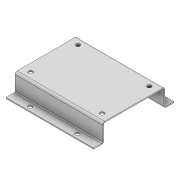
# Autodesk Inventor part: BaseMotor
Saved by Autodesk Inventor 2021 (Build 250183000, 183)
## iProperties
Created: 2021-08-18
Part Number: BaseMotor
Material: Generic
Document SubType Name: Sheet Metal
Designer: Santiago Suárez
Density: 1 g/cm^3
Sheet Metal Rule: Default_mm
Appearance: Default
Author: Santiago Suárez
Autodesk Inventor part; units mm, degrees
ref_plane "YZ Plane" through (0, 0, 0) normal (1, 0, 0) x (0, 1, 0)
ref_plane "XZ Plane" through (0, 0, 0) normal (0, 1, 0) x (-1, 0, 0)
ref_plane "XY Plane" through (0, 0, 0) normal (0, 0, 1) x (1, 0, 0)
sketch "Sketch1" plane through (0, 0, 0) normal (0, 1, 0) x (-1, 0, 0)
  line L0 (130, 92.5) -> (-130, 92.5)
  line L1 (-130, 92.5) -> (-130, -92.5)
  line L2 (-130, -92.5) -> (130, -92.5)
  line L3 (130, -92.5) -> (130, 92.5)
  point P0 (0, 0)
  dimension "d0" = 260
  dimension "d1" = 185
  dimension "d2" = 92.5
  dimension "d29" = 130
  measures "d0" distance of L0.start L0.end
  measures "d1" distance of L2.end L0.start
  measures "d2" distance from line of L0 point (0, 0)
  measures "d29" distance from line of L3 point (0, 0)
extrude "Plate1" add sketch "Sketch1" along normal blind 3.175
sketch "Sketch2" plane through (130, 3.175, 89.325) normal (0, 0, 1) x (1, 0, 0)
  line L0 (-260, 0) -> (0, 0)
  line L1 (0, 0) -> (0, 55)
  line L2 (0, 55) -> (-260, 55)
  line L3 (-260, 55) -> (-260, 0)
  constraints: 6 end point, 1 horizontal, 1 perpendicular, 1 vertical
edge flange "Flange1" height 55 angle 90 thickness 3.175 bend radius 3.175 thickness toward (0, 0, 1) relief straight relief width 3.175 relief depth 1.5875 edges at (0, 3.175, 92.5) wall of the first edge with corners at (-130, 3.175, 89.325) (130, 3.175, 89.325) (130, -51.825, 89.325) (-130, -51.825, 89.325)
bend "Bend1"
corner "Corner1"
sketch "Sketch3" plane through (-130, 3.175, -89.325) normal (0, 0, -1) x (-1, 0, 0)
  line L0 (-260, 0) -> (0, 0)
  line L1 (0, 0) -> (0, 55)
  line L2 (0, 55) -> (-260, 55)
  line L3 (-260, 55) -> (-260, 0)
  constraints: 6 end point, 1 horizontal, 1 perpendicular, 1 vertical
edge flange "Flange2" height 55 angle 90 thickness 3.175 bend radius 3.175 thickness toward (0, 0, -1) relief straight relief width 3.175 relief depth 1.5875 edges at (0, 3.175, -92.5) wall of the first edge with corners at (130, 3.175, -89.325) (-130, 3.175, -89.325) (-130, -51.825, -89.325) (130, -51.825, -89.325)
bend "Bend2"
corner "Corner2"
sketch "Sketch4" plane through (0, 3.175, 0) normal (0, 1, 0) x (1, 0, 0)
  line L0 (-106, -70) -> (106, -70)
  line L1 (106, -70) -> (106, 70)
  line L2 (106, 70) -> (-106, 70)
  line L3 (-106, 70) -> (-106, -70)
  line L4 (-130, -86.15) -> (-130, 86.15) projected
  point P0 (0, 0)
  dimension "d24" = 140
  dimension "d25" = 212
  dimension "d27" = 70
  dimension "d28" = 106
  constraints: 8 end point, 4 coincident, 2 parallel, 1 horizontal, 1 perpendicular
  measures "d24" distance of L2.end L0.start
  measures "d25" distance of L0.start L0.end
  measures "d27" distance from line of point (0, 0) L0
  measures "d28" distance from line of point (0, 0) L3
hole "Hole1" at (-106, 3.175, 70) at (-106, 3.175, -70) at (106, 3.175, 70) at (106, 3.175, -70) direction (0, -1, 0) diameter 12 depth 3.175
sketch "Sketch5" plane through (130, -48.65, -89.325) normal (0, -1, 0) x (1, 0, 0)
  line L0 (-260, 0) -> (0, 0)
  line L1 (0, 0) -> (0, 30)
  line L2 (0, 30) -> (-260, 30)
  line L3 (-260, 30) -> (-260, 0)
  constraints: 6 end point, 1 horizontal, 1 perpendicular, 1 vertical
edge flange "Flange3" height 30 angle 90 thickness 3.175 bend radius 3.175 thickness toward (0, -1, 0) relief straight relief width 3.175 relief depth 1.5875 edges at (0, -51.825, -89.325) wall of the first edge with corners at (-130, -48.65, -89.325) (130, -48.65, -89.325) (130, -48.65, -119.325) (-130, -48.65, -119.325)
bend "Bend3"
corner "Corner3"
sketch "Sketch6" plane through (-130, -48.65, 89.325) normal (0, -1, 0) x (1, 0, 0)
  line L0 (260, 0) -> (0, 0)
  line L1 (0, 0) -> (0, -30)
  line L2 (0, -30) -> (260, -30)
  line L3 (260, -30) -> (260, 0)
  constraints: 6 end point, 1 horizontal, 1 perpendicular, 1 vertical
edge flange "Flange4" height 30 angle 90 thickness 3.175 bend radius 3.175 thickness toward (0, -1, 0) relief straight relief width 3.175 relief depth 1.5875 edges at (0, -51.825, 89.325) wall of the first edge with corners at (130, -48.65, 89.325) (-130, -48.65, 89.325) (-130, -48.65, 119.325) (130, -48.65, 119.325)
bend "Bend4"
corner "Corner4"
sketch "Sketch7" plane through (-130, -48.65, 119.325) normal (0, 1, 0) x (1, 0, 0)
  line L0 (0, 23.65) -> (0, 0) projected
  line L1 (0, 11.825) -> (260, 11.825)
  line L2 (260, 0) -> (0, 0) projected
  line L3 (60, 0) -> (60, 24)
  line L4 (200, 0) -> (200, 24)
  line L5 (260, 23.65) -> (260, 0) projected
  point P0 (130, 119.325)
  point P1 (60, 11.825)
  point P2 (200, 11.825)
  dimension "d57" = 60
  dimension "d58" = 60
  constraints: 6 end point, 6 point on line, 1 horizontal, 1 midpoint, 1 perpendicular, 1 vertical
  measures "d57" distance between parallel lines of L4 L5
  measures "d58" distance between parallel lines of L3 L0
hole "Hole2" at (-70, -48.65, 107.5) at (70, -48.65, 107.5) direction (0, -1, 0) diameter 12 depth 3.175
mirror "Mirror1" about plane through (0, 0, 0) normal (0, 0, 1) of "Hole2"
equation "\"d28\" = 0.5 * d25"
equation "\"d35\" = Thickness"
equation "\"d64\" = Thickness"
equation "\"d3\" = Thickness"
equation "\"d4\" = BendReliefWidth"
equation "\"d5\" = BendReliefDepth"
equation "\"d6\" = MinimumRemnant"
equation "\"d7\" = TransitionRadius"
equation "\"d10\" = BendRadius"
equation "\"d11\" = CornerReliefSize"
equation "\"d12\" = GapSize"
equation "\"d13\" = JacobiRadiusSize"
equation "\"d14\" = BendReliefWidth"
equation "\"d15\" = BendReliefDepth"
equation "\"d16\" = MinimumRemnant"
equation "\"d17\" = TransitionRadius"
equation "\"d20\" = BendRadius"
equation "\"d21\" = CornerReliefSize"
equation "\"d22\" = GapSize"
equation "\"d23\" = JacobiRadiusSize"
equation "\"d37\" = BendReliefWidth"
equation "\"d38\" = BendReliefDepth"
equation "\"d39\" = MinimumRemnant"
equation "\"d40\" = TransitionRadius"
equation "\"d43\" = BendRadius"
equation "\"d44\" = CornerReliefSize"
equation "\"d45\" = GapSize"
equation "\"d46\" = JacobiRadiusSize"
equation "\"d47\" = BendReliefWidth"
equation "\"d48\" = BendReliefDepth"
equation "\"d49\" = MinimumRemnant"
equation "\"d50\" = TransitionRadius"
equation "\"d53\" = BendRadius"
equation "\"d54\" = CornerReliefSize"
equation "\"d55\" = GapSize"
equation "\"d56\" = JacobiRadiusSize"
equation "\"d2\" = 0.5 * d1"
equation "\"d29\" = 0.5 * d0"
equation "\"BendRadius\" = Thickness"
equation "\"BendReliefWidth\" = Thickness"
equation "\"BendReliefDepth\" = 0.5 * Thickness"
equation "\"CornerReliefSize\" = 4 * Thickness"
equation "\"MinimumRemnant\" = 2 * Thickness"
equation "\"TransitionRadius\" = BendRadius"
equation "\"JacobiRadiusSize\" = BendRadius"
equation "\"GapSize\" = Thickness"
equation "\"Thickness\" = 3.175"
body "Solid1"
